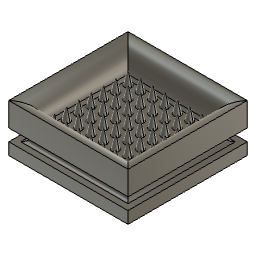
box final v2 (Autodesk Fusion 360 design; units mm, degrees)
Autodesk Fusion 360 part; units mm, degrees
sketch "Sketch1" plane through (0, 0, 0) normal (0, 0, 1) x (1, 0, 0)
  line L0 (0, 0) -> (50, 0)
  line L1 (50, 0) -> (50, 50)
  line L2 (50, 50) -> (0, 50)
  line L3 (0, 50) -> (0, 0)
  dimension "d1" = 50
  dimension "d2" = 50
  constraint horizontal L0
  constraint vertical L1
  constraint horizontal L2
  constraint vertical L3
  constraint coincident L0.start L3.end
  measures "d1" distance of L0.start L0.end
  measures "d2" distance of L0.start L2.end
extrude "Extrude1" add sketch "Sketch1" along normal blind 20 makes body 1
sketch "Sketch2" plane through (0, 0, 0) normal (0, -1, 0) x (1, 0, 0)
  line L0 (0, 0) -> (50, 0)
  line L1 (50, 0) -> (50, 20)
  line L2 (50, 20) -> (0, 20)
  line L3 (0, 20) -> (0, 0)
  line L4 (0, 10) -> (50, 10)
  line L5 (0, 5) -> (50, 5)
  constraint midpoint L3 L4.start
  constraint midpoint L1 L4.end
  constraint coincident L3 L5.start
  constraint coincident L1 L5.end
  constraint perpendicular L1 L5
sketch "Sketch3" plane through (50, 0, 0) normal (1, 0, 0) x (0, 1, 0)
  line L0 (0, 0) -> (50, 0)
  line L1 (50, 0) -> (50, 20)
  line L2 (50, 20) -> (0, 20)
  line L3 (0, 20) -> (0, 0)
  line L4 (0, 10) -> (50, 10)
  line L5 (0, 5) -> (50, 5)
  constraint midpoint L3 L4.start
  constraint midpoint L1 L4.end
  constraint coincident L3 L5.start
  constraint coincident L1 L5.end
  constraint perpendicular L1 L5
sketch "Sketch4" plane through (0, 50, 0) normal (0, 1, 0) x (-1, 0, 0)
  line L0 (-50, 0) -> (0, 0)
  line L1 (0, 0) -> (0, 20)
  line L2 (0, 20) -> (-50, 20)
  line L3 (-50, 20) -> (-50, 0)
  line L4 (-50, 10) -> (0, 10)
  line L5 (-50, 5) -> (0, 5)
  constraint midpoint L3 L4.start
  constraint midpoint L1 L4.end
  constraint coincident L3 L5.start
  constraint coincident L1 L5.end
  constraint perpendicular L1 L5
sketch "Sketch5" plane through (0, 0, 0) normal (-1, 0, 0) x (0, -1, 0)
  line L0 (-50, 0) -> (0, 0)
  line L1 (0, 0) -> (0, 20)
  line L2 (0, 20) -> (-50, 20)
  line L3 (-50, 20) -> (-50, 0)
  line L4 (-50, 10) -> (0, 10)
  line L5 (-50, 5) -> (0, 5)
  constraint midpoint L3 L4.start
  constraint midpoint L1 L4.end
  constraint coincident L3 L5.start
  constraint coincident L1 L5.end
  constraint perpendicular L1 L5
extrude "Extrude2" cut sketch "Sketch4" against normal blind 5 contours L1 L3 L4 L5 bodies 1
extrude "Extrude3" cut sketch "Sketch3" against normal blind 5 contours L1 L3 L4 L5 bodies 1
extrude "Extrude4" cut sketch "Sketch5" against normal blind 5 contours L1 L3 L4 L5 bodies 1
extrude "Extrude5" cut sketch "Sketch2" against normal blind 5 contours L1 L3 L4 L5 bodies 1
sketch "Sketch6" plane through (0, 0, 0) normal (0, 0, -1) x (1, 0, 0)
  line L0 (0, 0) -> (0, -50)
  line L1 (0, -50) -> (50, -50)
  line L2 (50, -50) -> (50, 0)
  line L3 (50, 0) -> (0, 0)
  line L4 (0, 0) -> (50, -50)
  line L5 (0, -50) -> (50, 0)
  circle A0 centre (25, -25) radius 12.5
  line L6 (42.5, -7.5) -> (7.5, -7.5)
  line L7 (7.5, -7.5) -> (7.5, -42.5)
  line L8 (7.5, -42.5) -> (42.5, -42.5)
  line L9 (42.5, -42.5) -> (42.5, -7.5)
  line L10 (42.5, -7.5) -> (7.5, -42.5) construction
  line L11 (7.5, -7.5) -> (42.5, -42.5) construction
  point P0 (25, -25)
  dimension "d14" = 35
  dimension "d15" = 35
  constraint coincident L0.start L3.end
  constraint coincident L1.end L2.start
  constraint coincident L0.end L1.start
  constraint coincident L2.end L3.start
  constraint midpoint L4 P0
  constraint horizontal L6
  constraint perpendicular L6 L7
  constraint parallel L6 L8
  constraint parallel L7 L9
  constraint coincident L10 P0
  constraint coincident L11 P0
  constraint coincident P0 A0.centre
  measures "d14" distance of L7.end L8.end
  measures "d15" distance of L6.end L7.end
extrude "Extrude6" cut sketch "Sketch6" against normal blind 2 contours L4 L5 A0 L6 | L4 L5 A0 L7 | L4 L5 A0 L8 | L4 L5 A0 L9 | L4 L5 A0 | L4 L5 A0 | L4 L5 A0 | L4 L5 A0 bodies 1
sketch "Sketch7" plane through (0, 0, 20) normal (0, 0, 1) x (-1, 0, 0)
  line L0 (0, -50) -> (0, 0)
  line L1 (0, 0) -> (-50, 0)
  line L2 (-50, 0) -> (-50, -50)
  line L3 (-50, -50) -> (0, -50)
  line L4 (-42.5, -7.5) -> (-7.5, -7.5)
  line L5 (-7.5, -7.5) -> (-7.5, -42.5)
  line L6 (-7.5, -42.5) -> (-42.5, -42.5)
  line L7 (-42.5, -42.5) -> (-42.5, -7.5)
  line L8 (-45, -5) -> (-5, -5)
  line L9 (-5, -5) -> (-5, -45)
  line L10 (-5, -45) -> (-45, -45)
  line L11 (-45, -45) -> (-45, -5)
  point P0 (-25, -25)
  point P1 (-25, -25)
  dimension "d19" = 35
  dimension "d21" = 40
  constraint horizontal L4
  constraint perpendicular L4 L5
  constraint parallel L4 L6
  constraint parallel L5 L7
  constraint horizontal L8
  constraint perpendicular L8 L9
  constraint parallel L8 L10
  constraint parallel L9 L11
  constraint coincident P1 P0
  measures "d19" distance of L4.end L5.end
  measures "d21" distance of L8.end L9.end
extrude "Extrude7" cut sketch "Sketch7" against normal blind 5 contours L4 L5 L6 L7 bodies 1
sketch "Sketch8" plane through (0, 0, 15) normal (0, 0, 1) x (-1, 0, 0)
  line L0 (-42.5, -42.5) -> (-7.5, -42.5)
  line L1 (-7.5, -42.5) -> (-7.5, -7.5)
  line L2 (-7.5, -7.5) -> (-42.5, -7.5)
  line L3 (-42.5, -7.5) -> (-42.5, -42.5)
extrude "Extrude8" cut sketch "Sketch8" against normal blind 5 bodies 1
sketch "Sketch9" plane through (0, 42.5, 0) normal (0, -1, 0) x (1, 0, 0)
  line L0 (42.5, 20) -> (7.5, 20)
  line L1 (7.5, 20) -> (7.5, 10)
  line L2 (7.5, 10) -> (42.5, 10)
  line L3 (42.5, 10) -> (42.5, 20)
  line L4 (7.5, 10) -> (10.5, 10)
  line L5 (9, 16.7584) -> (9, 10)
  spline S0 degree 2 poles (9, 15.0688) (9.3306, 15.0688) (10.2617, 11.0737) (10.5, 10) knots 0 0 0 0.446246 0.531047 0.531047 0.531047 weights 1 1.348069 1.066144 1
  dimension "d26" = 3
  constraint coincident L1.end L2.start
  constraint perpendicular L1 L4
  constraint midpoint L4 L5.end
  constraint perpendicular L4 L5
  constraint coincident L5 S0.start
  measures "d26" distance of L1.end L4.end
revolve "Revolve1" add sketch "Sketch9" angle 360 about axis through (9, 42.5, 16.7584) along (0, 0, -1) separate body contours L2 L4 L5 S0 makes body 2
move_body "Move1" bodies 2 to x (1, 0, 0) y (0, 1, 0) z (0, 0, 1) at (0.5, -2, 0)
pattern_linear "R-Pattern1" count 7 spacing 5.1667 along (0, -1, 0) count 7 spacing 5.1667 along (1, 0, 0) of bodies 2 makes body 3 at (10.2232, 34.2338, 10.8225) makes body 4 at (10.2232, 29.0671, 10.8225) makes body 5 at (10.2232, 23.9005, 10.8225) makes body 6 at (10.2232, 18.7338, 10.8225) makes body 7 at (10.2232, 13.5671, 10.8225) makes body 8 at (10.2232, 8.4005, 10.8225) makes body 9 at (15.3898, 39.4005, 10.8225) makes body 10 at (15.3898, 34.2338, 10.8225) makes body 11 at (15.3898, 29.0671, 10.8225) makes body 12 at (15.3898, 23.9005, 10.8225) makes body 13 at (15.3898, 18.7338, 10.8225) makes body 14 at (15.3898, 13.5671, 10.8225) makes body 15 at (15.3898, 8.4005, 10.8225) makes body 16 at (20.5565, 41.5995, 10.8225) makes body 17 at (20.5565, 34.2338, 10.8225) makes body 18 at (20.5565, 29.0671, 10.8225) makes body 19 at (20.5565, 23.9005, 10.8225) makes body 20 at (20.5565, 18.7338, 10.8225) makes body 21 at (20.5565, 15.7662, 10.8225) makes body 22 at (20.5565, 8.4005, 10.8225) makes body 23 at (25.7232, 39.4005, 10.8225) makes body 24 at (25.7232, 34.2338, 10.8225) makes body 25 at (25.7232, 29.0671, 10.8225) makes body 26 at (25.7232, 23.9005, 10.8225) makes body 27 at (25.7232, 18.7338, 10.8225) makes body 28 at (25.7232, 13.5671, 10.8225) makes body 29 at (25.7232, 8.4005, 10.8225) makes body 30 at (30.8898, 39.4005, 10.8225) makes body 31 at (30.8898, 34.2338, 10.8225) makes body 32 at (30.8898, 29.0671, 10.8225) makes body 33 at (30.8898, 23.9005, 10.8225) makes body 34 at (30.8898, 20.9329, 10.8225) makes body 35 at (30.8898, 13.5671, 10.8225) makes body 36 at (30.8898, 8.4005, 10.8225) makes body 37 at (36.0565, 39.4005, 10.8225) makes body 38 at (36.0565, 34.2338, 10.8225) makes body 39 at (36.0565, 29.0671, 10.8225) makes body 40 at (36.0565, 26.0995, 10.8225) makes body 41 at (36.0565, 18.7338, 10.8225) makes body 42 at (36.0565, 13.5671, 10.8225) makes body 43 at (36.0565, 8.4005, 10.8225) makes body 44 at (41.2232, 41.5995, 10.8225) makes body 45 at (41.2232, 34.2338, 10.8225) makes body 46 at (41.2232, 29.0671, 10.8225) makes body 47 at (41.2232, 26.0995, 10.8225) makes body 48 at (41.2232, 18.7338, 10.8225) makes body 49 at (41.2232, 13.5671, 10.8225) makes body 50 at (41.2232, 8.4005, 10.8225)
fillet "Fillet1" radius 8 4 edges at (7.5, 25, 20) (25, 42.5, 20) (42.5, 25, 20) (25, 7.5, 20) on bodies 1
combine "Combine1" operation add target body 1 tool bodies 2 3 4 5 6 7 8 9 10 11 12 13 14 15 16 17 18 19 20 21 22 24 23 25 26 27 28 29 30 31 32 33 34 35 36 37 38 39 40 41 42 43 44 45 46 47 48 49 50
fillet "Fillet2" radius 2.5 8 edges at (5, 25, 5) (25, 45, 5) (5, 25, 10) (25, 45, 10) (25, 5, 5) (25, 5, 10) (45, 25, 5) (45, 25, 10) on bodies 1
